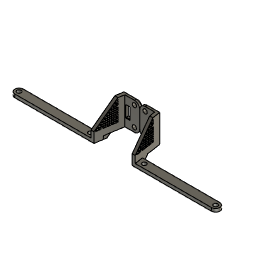
BLTouch_Halter_standardv4 (Autodesk Fusion 360 design; units mm, degrees)
Autodesk Fusion 360 part; units mm, degrees
note: some values were not read from the file. Chosen so that the rebuilt part matches the saved one: which face or edge a step refers to.
(part 1 of 2)
sketch "Skizze1" plane through (0, 0, 0) normal (0, 0, 1) x (1, 0, 0)
  line L0 (115.7718, 101.7058) -> (145.7718, 101.7066) construction
  line L1 (93.7718, 101.7055) -> (63.7718, 101.7055) construction
  line L2 (63.7718, 101.7055) -> (71.2754, 51.2606) construction
  line L3 (145.7718, 101.7066) -> (138.2754, 51.2606) construction
  circle A0 centre (63.7718, 101.7055) radius 1.5
  circle A1 centre (145.7718, 101.7066) radius 1.5
  circle A2 centre (138.2754, 51.2606) radius 2
  circle A3 centre (71.2754, 51.2606) radius 2
  circle A4 centre (93.7718, 101.7055) radius 1.5
  circle A5 centre (115.7718, 101.7058) radius 1.5
  line L4 (145.7718, 101.7066) -> (108.2713, 130.0389) construction
  line L5 (108.2713, 130.0389) -> (101.2713, 130.0389) construction
  line L6 (101.2713, 130.0389) -> (63.7718, 101.7055) construction
  circle A6 centre (101.2713, 130.0389) radius 1
  circle A7 centre (108.2713, 130.0389) radius 1
  line L7 (103.2307, 127.4457) -> (106.3121, 127.4456)
  line L8 (71.2754, 51.2606) -> (71.2754, 46.4951) construction
  line L9 (71.2754, 51.2606) -> (69.2754, 51.2606) construction
  line L10 (71.2754, 51.2606) -> (138.2754, 51.2606) construction
  line L11 (143.9247, 55.2606) -> (146.8968, 75.2606)
  line L12 (71.2754, 47.2606) -> (138.2754, 47.2606)
  arc A8 (138.8634, 55.2171) -> (138.2754, 55.2606) centre (138.2754, 51.2606) ccw
  line L13 (138.2754, 55.2606) -> (71.2754, 55.2606)
  arc A9 (71.2754, 55.2606) -> (71.2754, 47.2606) centre (71.2754, 51.2606) ccw
  line L14 (71.2754, 51.2606) -> (138.2754, 51.2606) construction
  line L15 (138.2754, 55.2606) -> (143.9247, 55.2606)
  line L16 (146.8968, 75.2606) -> (163.4839, 75.2606)
  line L17 (163.4839, 75.2606) -> (163.4839, 72.2606)
  line L18 (163.4839, 72.2606) -> (149.4839, 72.2606)
  line L19 (149.4839, 72.2606) -> (145.5714, 47.2606)
  line L20 (138.2754, 47.2606) -> (145.5714, 47.2606)
  line L21 (143.9247, 55.2606) -> (142.7359, 47.2606) construction
  line L22 (149.4839, 72.2606) -> (149.4839, 75.2606) construction
  dimension "d8" = 30
  dimension "d9" = 30
  dimension "d11" = 3
  dimension "d12" = 3
  dimension "d13" = 4
  dimension "d14" = 4
  dimension "d16" = 51
  dimension "d17" = 81.546
  dimension "d19" = 81.5
  dimension "d28" = 3
  dimension "d29" = 3
  dimension "d30" = 47
  dimension "d31" = 47
  dimension "d33" = 7
  dimension "d34" = 2
  dimension "d35" = 2
  dimension "d36" = 37.1
  dimension "d37" = 142.9
  dimension "d38" = 37.1
  dimension "d39" = 67
  dimension "d69" = 8
  dimension "d71" = 5
  dimension "d73" = 24
  dimension "d74" = 3
  dimension "d75" = 3
  dimension "d76" = 14
  constraint horizontal L1
  constraint coincident L1.end L2.start
  constraint coincident L0.end L3.start
  constraint coincident L3.end A2.centre
  constraint coincident L2.end A3.centre
  constraint coincident L1.start A4.centre
  constraint coincident L0.start A5.centre
  constraint horizontal L5
  constraint coincident L5.end L6.start
  constraint coincident L4.end L5.start
  constraint perpendicular L8 L9
  constraint coincident A3 L9.end
  constraint perpendicular L8 L10
  constraint parallel L3 L11
  constraint tangent L12 A8
  constraint tangent A8 L13
  constraint parallel L12 L13
  constraint tangent L13 A9
  constraint tangent L12 A9
  constraint parallel L10 L14
  constraint tangent A8 L15
  constraint coincident L3 A8.start
  constraint horizontal L16
  constraint perpendicular L16 L17
  constraint perpendicular L17 L18
  constraint parallel L12 L20
  constraint coincident L20 L21.end
  constraint parallel L11 L21
  constraint coincident L16 L22.end
  constraint perpendicular L16 L22
  measures "d8" distance of L0.start L0.end
  measures "d9" distance of L1.start L1.end
  measures "d11" diameter of A0
  measures "d12" diameter of A1
  measures "d13" diameter of A2
  measures "d14" diameter of A3
  measures "d16" distance of L3.end L0.end
  measures "d17" angle of L0 L3
  measures "d28" diameter of A4
  measures "d29" diameter of A5
  measures "d30" distance of L0.end L4.end
  measures "d31" distance of L5.end L1.end
  measures "d33" distance of L4.end L5.end
  measures "d34" diameter of A6
  measures "d35" diameter of A7
  measures "d39" distance of L2.end L3.end
  measures "d69" diameter of A8
  measures "d71" distance of L3 L11
  measures "d73" vertical distance of L3.end L11.end
  measures "d74" distance of L16.end L17.end
  measures "d75" distance of L11 L18.end
  measures "d76" distance of L17.end L18.end
extrude "Extrusion11" add sketch "Skizze1" along normal blind 3 contours L11 L12 L13 A9 L15 L16 L17 L18 L19 L20 makes body 1
sketch "Skizze8" plane through (0, 0, 3) normal (0, 0, 1) x (-1, 0, 0)
  circle A0 centre (-138.2754, -51.2606) radius 2
  circle A1 centre (-71.2754, -51.2606) radius 2
  line L0 (-143.9247, -55.2606) -> (-71.2754, -55.2606)
  arc A2 (-71.2754, -55.2606) -> (-71.2754, -47.2606) centre (-71.2754, -51.2606) ccw
  line L1 (-71.2754, -47.2606) -> (-145.5714, -47.2606)
  line L2 (-145.5714, -47.2606) -> (-149.4839, -72.2606)
  line L3 (-149.4839, -72.2606) -> (-163.4839, -72.2606)
  line L4 (-163.4839, -72.2606) -> (-163.4839, -75.2606)
  line L5 (-163.4839, -75.2606) -> (-146.8968, -75.2606)
  line L6 (-146.8968, -75.2606) -> (-143.9247, -55.2606)
  line L7 (-143.9247, -55.2606) -> (-142.7359, -47.2606)
  line L8 (-143.9247, -55.2606) -> (-146.8968, -75.2606)
  line L9 (-163.4839, -75.2606) -> (-163.4839, -72.2606)
  line L10 (-149.4839, -72.2606) -> (-163.4839, -72.2606)
  line L11 (-149.4839, -72.2606) -> (-145.5714, -47.2606)
  line L12 (-145.5714, -47.2606) -> (-142.7359, -47.2606)
  constraint coincident L0.start L6.end
  constraint coincident L1 L7.end
  constraint parallel L6 L7
  constraint coincident L5.end L6.start
  constraint coincident L4.end L5.start
  constraint coincident L3.end L4.start
  constraint coincident L2.end L3.start
  constraint coincident L1.end L2.start
extrude "Extrusion12" add sketch "Skizze8" along normal blind 23 contours L1 L2 L3 L4 L5 L6 L7 L8 L9 L10 L11 L12 bodies 1
sketch "Skizze10" plane through (0, 75.2606, 0) normal (0, 1, 0) x (-1, 0, 0)
  line L0 (-163.4839, 0) -> (-146.8968, 0)
  line L1 (-146.8968, 0) -> (-146.8968, 26)
  line L2 (-146.8968, 26) -> (-163.4839, 26)
  line L3 (-163.4839, 26) -> (-163.4839, 0)
  line L4 (-158.4839, 26) -> (-158.4839, 0) construction
  line L5 (-146.8968, 13) -> (-163.4839, 13) construction
  circle A0 centre (-158.4839, 22) radius 2
  circle A1 centre (-158.4839, 4) radius 2
  point P0 (-158.4839, 13)
  dimension "d82" = 4
  dimension "d83" = 9
  dimension "d111" = 5
  dimension "d112" = 9
  constraint midpoint L1 L5.start
  constraint midpoint L3 L5.end
  constraint coincident L4 A0.centre
  constraint coincident L4 A1.centre
  measures "d82" diameter of A0
  measures "d83" distance of P0 A0.centre
  measures "d111" distance of L3 L4
  measures "d112" distance of L5 A1.centre
extrude "Extrusion13" cut sketch "Skizze10" against normal blind 6 contours A0 | A1 bodies 1
fillet "Abrundung1" radius 5 2 edges at (163.4839, 73.7606, 26) (163.4839, 73.7606, 0) on bodies 1
chamfer "Fase1" distance 19.5 angle 45 1 edges at (144.1537, 47.2606, 26) on bodies 1
sketch "Skizze12" plane through (132.7809, -19.7314, 0) normal (-0.989138, 0.146987, 0) x (-0.146987, -0.989138, 0)
  line L0 (-67.7276, 6.5) -> (-87.4417, 26)
  line L1 (-87.4417, 26) -> (-96.035, 26)
  line L2 (-96.035, 26) -> (-96.035, 0)
  line L3 (-96.035, 0) -> (-75.8154, 0)
  line L4 (-75.8154, 0) -> (-75.8154, 3)
  line L5 (-75.8154, 3) -> (-67.7276, 3)
  line L6 (-67.7276, 3) -> (-67.7276, 6.5)
  line L7 (-75.8154, 3) -> (-96.035, 3)
  line L8 (-96.035, 26) -> (-96.035, 3)
  line L9 (-96.035, 26) -> (-87.4417, 26)
  line L10 (-87.4417, 26) -> (-67.7276, 6.5)
  line L11 (-67.7276, 3) -> (-67.7276, 6.5)
  line L12 (-67.7276, 3) -> (-75.8154, 3)
  line L13 (-71.9936, 6) -> (-75.3099, 6)
  line L14 (-75.3099, 6) -> (-87.9801, 6)
  line L15 (-87.9801, 21.8129) -> (-87.9801, 6)
  line L16 (-87.6401, 24.2897) -> (-69.5914, 6.437)
  line L17 (-87.9801, 21.8129) -> (-87.9801, 24.2897)
  line L18 (-71.9936, 6) -> (-69.5914, 6)
  line L19 (-69.5914, 6) -> (-69.5914, 6.437)
  line L20 (-87.9801, 24.2897) -> (-87.9472, 24.2897)
  line L21 (-87.9472, 24.2897) -> (-87.6401, 24.2897)
  line L22 (-75.8154, 1.0103) -> (-75.3808, 0.584)
  line L23 (-74.6486, 3) -> (-73.8108, 2.1712)
  line L24 (-79.7376, 15.0605) -> (-80.8491, 14.7474)
  line L25 (-80.8491, 14.7474) -> (-81.1336, 13.6283)
  line L26 (-81.1336, 13.6283) -> (-80.3068, 12.8223)
  line L27 (-80.3068, 12.8223) -> (-79.1953, 13.1355)
  line L28 (-79.1953, 13.1355) -> (-78.9108, 14.2545)
  line L29 (-78.9108, 14.2545) -> (-79.7376, 15.0605)
  line L30 (-97.415, 14.964) -> (-98.5265, 14.6509)
  line L31 (-98.5265, 14.6509) -> (-98.811, 13.5318)
  line L32 (-98.811, 13.5318) -> (-97.9842, 12.7258)
  line L33 (-97.9842, 12.7258) -> (-96.8727, 13.0389)
  line L34 (-96.5882, 14.158) -> (-97.415, 14.964)
  line L35 (-96.8727, 13.0389) -> (-96.5882, 14.158)
  line L36 (-95.6377, 13.2059) -> (-96.7491, 12.8928)
  line L37 (-96.7491, 12.8928) -> (-97.0336, 11.7737)
  line L38 (-97.0336, 11.7737) -> (-96.2068, 10.9677)
  line L39 (-96.2068, 10.9677) -> (-95.0953, 11.2808)
  line L40 (-94.8108, 12.3999) -> (-95.6377, 13.2059)
  line L41 (-95.0953, 11.2808) -> (-94.8108, 12.3999)
  line L42 (-93.8603, 11.4478) -> (-94.9717, 11.1347)
  line L43 (-94.9717, 11.1347) -> (-95.2563, 10.0156)
  line L44 (-95.2563, 10.0156) -> (-94.4294, 9.2096)
  line L45 (-94.4294, 9.2096) -> (-93.3179, 9.5228)
  line L46 (-93.0334, 10.6418) -> (-93.8603, 11.4478)
  line L47 (-93.3179, 9.5228) -> (-93.0334, 10.6418)
  line L48 (-92.0829, 9.6897) -> (-93.1943, 9.3766)
  line L49 (-93.1943, 9.3766) -> (-93.4789, 8.2575)
  line L50 (-93.4789, 8.2575) -> (-92.652, 7.4516)
  line L51 (-92.652, 7.4516) -> (-91.5405, 7.7647)
  line L52 (-91.256, 8.8838) -> (-92.0829, 9.6897)
  line L53 (-91.5405, 7.7647) -> (-91.256, 8.8838)
  line L54 (-90.3055, 7.9316) -> (-91.4169, 7.6185)
  line L55 (-91.4169, 7.6185) -> (-91.7015, 6.4994)
  line L56 (-91.7015, 6.4994) -> (-90.8746, 5.6935)
  line L57 (-90.8746, 5.6935) -> (-89.7631, 6.0066)
  line L58 (-89.4786, 7.1257) -> (-90.3055, 7.9316)
  line L59 (-89.7631, 6.0066) -> (-89.4786, 7.1257)
  line L60 (-88.5281, 6.1736) -> (-89.6395, 5.8604)
  line L61 (-89.6395, 5.8604) -> (-89.9241, 4.7414)
  line L62 (-89.9241, 4.7414) -> (-89.0972, 3.9354)
  line L63 (-89.0972, 3.9354) -> (-87.9858, 4.2485)
  line L64 (-87.7012, 5.3676) -> (-88.5281, 6.1736)
  line L65 (-87.9858, 4.2485) -> (-87.7012, 5.3676)
  line L66 (-86.7507, 4.4155) -> (-87.8621, 4.1024)
  line L67 (-87.8621, 4.1024) -> (-88.1467, 2.9833)
  line L68 (-88.1467, 2.9833) -> (-87.3198, 2.1773)
  line L69 (-87.3198, 2.1773) -> (-86.2084, 2.4904)
  line L70 (-85.9238, 3.6095) -> (-86.7507, 4.4155)
  line L71 (-86.2084, 2.4904) -> (-85.9238, 3.6095)
  line L72 (-84.9733, 2.6574) -> (-86.0847, 2.3443)
  line L73 (-86.0847, 2.3443) -> (-86.3693, 1.2252)
  line L74 (-86.3693, 1.2252) -> (-85.5424, 0.4192)
  line L75 (-85.5424, 0.4192) -> (-84.431, 0.7323)
  line L76 (-84.1464, 1.8514) -> (-84.9733, 2.6574)
  line L77 (-84.431, 0.7323) -> (-84.1464, 1.8514)
  line L78 (-83.1959, 0.8993) -> (-84.3073, 0.5862)
  line L79 (-84.3073, 0.5862) -> (-84.5919, -0.5329)
  line L80 (-84.5919, -0.5329) -> (-83.765, -1.3389)
  line L81 (-83.765, -1.3389) -> (-82.6536, -1.0258)
  line L82 (-82.369, 0.0933) -> (-83.1959, 0.8993)
  line L83 (-82.6536, -1.0258) -> (-82.369, 0.0933)
  line L84 (-81.4185, -0.8588) -> (-82.5299, -1.1719)
  line L85 (-82.5299, -1.1719) -> (-82.8145, -2.291)
  line L86 (-82.8145, -2.291) -> (-81.9876, -3.097)
  line L87 (-81.9876, -3.097) -> (-80.8762, -2.7839)
  line L88 (-80.5916, -1.6648) -> (-81.4185, -0.8588)
  line L89 (-80.8762, -2.7839) -> (-80.5916, -1.6648)
  line L90 (-79.6411, -2.6169) -> (-80.7526, -2.93)
  line L91 (-80.7526, -2.93) -> (-81.0371, -4.0491)
  line L92 (-81.0371, -4.0491) -> (-80.2102, -4.8551)
  line L93 (-80.2102, -4.8551) -> (-79.0988, -4.5419)
  line L94 (-78.8142, -3.4229) -> (-79.6411, -2.6169)
  line L95 (-79.0988, -4.5419) -> (-78.8142, -3.4229)
  line L96 (-95.657, 16.7414) -> (-96.7684, 16.4283)
  line L97 (-96.7684, 16.4283) -> (-97.053, 15.3092)
  line L98 (-97.053, 15.3092) -> (-96.2261, 14.5032)
  line L99 (-96.2261, 14.5032) -> (-95.1146, 14.8163)
  line L100 (-94.8301, 15.9354) -> (-95.657, 16.7414)
  line L101 (-95.1146, 14.8163) -> (-94.8301, 15.9354)
  line L102 (-93.8796, 14.9833) -> (-94.991, 14.6702)
  line L103 (-94.991, 14.6702) -> (-95.2756, 13.5511)
  line L104 (-95.2756, 13.5511) -> (-94.4487, 12.7451)
  line L105 (-94.4487, 12.7451) -> (-93.3372, 13.0582)
  line L106 (-93.0527, 14.1773) -> (-93.8796, 14.9833)
  line L107 (-93.3372, 13.0582) -> (-93.0527, 14.1773)
  line L108 (-92.1022, 13.2252) -> (-93.2136, 12.9121)
  line L109 (-93.2136, 12.9121) -> (-93.4982, 11.793)
  line L110 (-93.4982, 11.793) -> (-92.6713, 10.987)
  line L111 (-92.6713, 10.987) -> (-91.5598, 11.3001)
  line L112 (-91.2753, 12.4192) -> (-92.1022, 13.2252)
  line L113 (-91.5598, 11.3001) -> (-91.2753, 12.4192)
  line L114 (-90.3248, 11.4671) -> (-91.4362, 11.154)
  line L115 (-91.4362, 11.154) -> (-91.7208, 10.0349)
  line L116 (-91.7208, 10.0349) -> (-90.8939, 9.2289)
  line L117 (-90.8939, 9.2289) -> (-89.7825, 9.5421)
  line L118 (-89.4979, 10.6612) -> (-90.3248, 11.4671)
  line L119 (-89.7825, 9.5421) -> (-89.4979, 10.6612)
  line L120 (-88.5474, 9.709) -> (-89.6588, 9.3959)
  line L121 (-89.6588, 9.3959) -> (-89.9434, 8.2768)
  line L122 (-89.9434, 8.2768) -> (-89.1165, 7.4709)
  line L123 (-89.1165, 7.4709) -> (-88.0051, 7.784)
  line L124 (-87.7205, 8.9031) -> (-88.5474, 9.709)
  line L125 (-88.0051, 7.784) -> (-87.7205, 8.9031)
  line L126 (-86.77, 7.951) -> (-87.8814, 7.6378)
  line L127 (-87.8814, 7.6378) -> (-88.166, 6.5187)
  line L128 (-88.166, 6.5187) -> (-87.3391, 5.7128)
  line L129 (-87.3391, 5.7128) -> (-86.2277, 6.0259)
  line L130 (-85.9431, 7.145) -> (-86.77, 7.951)
  line L131 (-86.2277, 6.0259) -> (-85.9431, 7.145)
  line L132 (-84.9926, 6.1929) -> (-86.104, 5.8798)
  line L133 (-86.104, 5.8798) -> (-86.3886, 4.7607)
  line L134 (-86.3886, 4.7607) -> (-85.5617, 3.9547)
  line L135 (-85.5617, 3.9547) -> (-84.4503, 4.2678)
  line L136 (-84.1657, 5.3869) -> (-84.9926, 6.1929)
  line L137 (-84.4503, 4.2678) -> (-84.1657, 5.3869)
  line L138 (-83.2152, 4.4348) -> (-84.3266, 4.1217)
  line L139 (-84.3266, 4.1217) -> (-84.6112, 3.0026)
  line L140 (-84.6112, 3.0026) -> (-83.7843, 2.1966)
  line L141 (-83.7843, 2.1966) -> (-82.6729, 2.5097)
  line L142 (-82.3883, 3.6288) -> (-83.2152, 4.4348)
  line L143 (-82.6729, 2.5097) -> (-82.3883, 3.6288)
  line L144 (-81.4378, 2.6767) -> (-82.5493, 2.3636)
  line L145 (-82.5493, 2.3636) -> (-82.8338, 1.2445)
  line L146 (-82.8338, 1.2445) -> (-82.0069, 0.4385)
  line L147 (-82.0069, 0.4385) -> (-80.8955, 0.7516)
  line L148 (-80.6109, 1.8707) -> (-81.4378, 2.6767)
  line L149 (-80.8955, 0.7516) -> (-80.6109, 1.8707)
  line L150 (-79.6604, 0.9186) -> (-80.7719, 0.6055)
  line L151 (-80.7719, 0.6055) -> (-81.0564, -0.5136)
  line L152 (-81.0564, -0.5136) -> (-80.2295, -1.3196)
  line L153 (-80.2295, -1.3196) -> (-79.1181, -1.0065)
  line L154 (-78.8335, 0.1126) -> (-79.6604, 0.9186)
  line L155 (-79.1181, -1.0065) -> (-78.8335, 0.1126)
  line L156 (-77.883, -0.8395) -> (-78.9945, -1.1526)
  line L157 (-78.9945, -1.1526) -> (-79.279, -2.2717)
  line L158 (-79.279, -2.2717) -> (-78.4521, -3.0777)
  line L159 (-78.4521, -3.0777) -> (-77.3407, -2.7646)
  line L160 (-77.0561, -1.6455) -> (-77.883, -0.8395)
  line L161 (-77.3407, -2.7646) -> (-77.0561, -1.6455)
  line L162 (-93.8989, 18.5188) -> (-95.0103, 18.2057)
  line L163 (-95.0103, 18.2057) -> (-95.2949, 17.0866)
  line L164 (-95.2949, 17.0866) -> (-94.468, 16.2806)
  line L165 (-94.468, 16.2806) -> (-93.3565, 16.5937)
  line L166 (-93.072, 17.7128) -> (-93.8989, 18.5188)
  line L167 (-93.3565, 16.5937) -> (-93.072, 17.7128)
  line L168 (-92.1215, 16.7607) -> (-93.2329, 16.4476)
  line L169 (-93.2329, 16.4476) -> (-93.5175, 15.3285)
  line L170 (-93.5175, 15.3285) -> (-92.6906, 14.5225)
  line L171 (-92.6906, 14.5225) -> (-91.5792, 14.8356)
  line L172 (-91.2946, 15.9547) -> (-92.1215, 16.7607)
  line L173 (-91.5792, 14.8356) -> (-91.2946, 15.9547)
  line L174 (-90.3441, 15.0026) -> (-91.4555, 14.6895)
  line L175 (-91.4555, 14.6895) -> (-91.7401, 13.5704)
  line L176 (-91.7401, 13.5704) -> (-90.9132, 12.7644)
  line L177 (-90.9132, 12.7644) -> (-89.8018, 13.0775)
  line L178 (-89.5172, 14.1966) -> (-90.3441, 15.0026)
  line L179 (-89.8018, 13.0775) -> (-89.5172, 14.1966)
  line L180 (-88.5667, 13.2445) -> (-89.6781, 12.9314)
  line L181 (-89.6781, 12.9314) -> (-89.9627, 11.8123)
  line L182 (-89.9627, 11.8123) -> (-89.1358, 11.0063)
  line L183 (-89.1358, 11.0063) -> (-88.0244, 11.3195)
  line L184 (-87.7398, 12.4385) -> (-88.5667, 13.2445)
  line L185 (-88.0244, 11.3195) -> (-87.7398, 12.4385)
  line L186 (-86.7893, 11.4864) -> (-87.9007, 11.1733)
  line L187 (-87.9007, 11.1733) -> (-88.1853, 10.0542)
  line L188 (-88.1853, 10.0542) -> (-87.3584, 9.2483)
  line L189 (-87.3584, 9.2483) -> (-86.247, 9.5614)
  line L190 (-85.9624, 10.6805) -> (-86.7893, 11.4864)
  line L191 (-86.247, 9.5614) -> (-85.9624, 10.6805)
  line L192 (-85.0119, 9.7283) -> (-86.1233, 9.4152)
  line L193 (-86.1233, 9.4152) -> (-86.4079, 8.2961)
  line L194 (-86.4079, 8.2961) -> (-85.581, 7.4902)
  line L195 (-85.581, 7.4902) -> (-84.4696, 7.8033)
  line L196 (-84.185, 8.9224) -> (-85.0119, 9.7283)
  line L197 (-84.4696, 7.8033) -> (-84.185, 8.9224)
  line L198 (-83.2345, 7.9703) -> (-84.3459, 7.6571)
  line L199 (-84.3459, 7.6571) -> (-84.6305, 6.5381)
  line L200 (-84.6305, 6.5381) -> (-83.8036, 5.7321)
  line L201 (-83.8036, 5.7321) -> (-82.6922, 6.0452)
  line L202 (-82.4076, 7.1643) -> (-83.2345, 7.9703)
  line L203 (-82.6922, 6.0452) -> (-82.4076, 7.1643)
  line L204 (-81.4571, 6.2122) -> (-82.5686, 5.8991)
  line L205 (-82.5686, 5.8991) -> (-82.8531, 4.78)
  line L206 (-82.8531, 4.78) -> (-82.0262, 3.974)
  line L207 (-82.0262, 3.974) -> (-80.9148, 4.2871)
  line L208 (-80.6302, 5.4062) -> (-81.4571, 6.2122)
  line L209 (-80.9148, 4.2871) -> (-80.6302, 5.4062)
  line L210 (-79.6797, 4.4541) -> (-80.7912, 4.141)
  line L211 (-80.7912, 4.141) -> (-81.0757, 3.0219)
  line L212 (-81.0757, 3.0219) -> (-80.2488, 2.2159)
  line L213 (-80.2488, 2.2159) -> (-79.1374, 2.529)
  line L214 (-78.8528, 3.6481) -> (-79.6797, 4.4541)
  line L215 (-79.1374, 2.529) -> (-78.8528, 3.6481)
  line L216 (-77.9023, 2.696) -> (-79.0138, 2.3829)
  line L217 (-79.0138, 2.3829) -> (-79.2983, 1.2638)
  line L218 (-79.2983, 1.2638) -> (-78.4714, 0.4578)
  line L219 (-78.4714, 0.4578) -> (-77.36, 0.7709)
  line L220 (-77.0755, 1.89) -> (-77.9023, 2.696)
  line L221 (-77.36, 0.7709) -> (-77.0755, 1.89)
  line L222 (-76.1249, 0.9379) -> (-77.2364, 0.6248)
  line L223 (-77.2364, 0.6248) -> (-77.5209, -0.4943)
  line L224 (-77.5209, -0.4943) -> (-76.6941, -1.3003)
  line L225 (-76.6941, -1.3003) -> (-75.5826, -0.9872)
  line L226 (-75.2981, 0.1319) -> (-76.1249, 0.9379)
  line L227 (-75.5826, -0.9872) -> (-75.2981, 0.1319)
  line L228 (-92.1408, 20.2962) -> (-93.2522, 19.9831)
  line L229 (-93.2522, 19.9831) -> (-93.5368, 18.864)
  line L230 (-93.5368, 18.864) -> (-92.7099, 18.058)
  line L231 (-92.7099, 18.058) -> (-91.5985, 18.3711)
  line L232 (-91.3139, 19.4902) -> (-92.1408, 20.2962)
  line L233 (-91.5985, 18.3711) -> (-91.3139, 19.4902)
  line L234 (-90.3634, 18.5381) -> (-91.4748, 18.225)
  line L235 (-91.4748, 18.225) -> (-91.7594, 17.1059)
  line L236 (-91.7594, 17.1059) -> (-90.9325, 16.2999)
  line L237 (-90.9325, 16.2999) -> (-89.8211, 16.613)
  line L238 (-89.5365, 17.7321) -> (-90.3634, 18.5381)
  line L239 (-89.8211, 16.613) -> (-89.5365, 17.7321)
  line L240 (-88.586, 16.78) -> (-89.6974, 16.4669)
  line L241 (-89.6974, 16.4669) -> (-89.982, 15.3478)
  line L242 (-89.982, 15.3478) -> (-89.1551, 14.5418)
  line L243 (-89.1551, 14.5418) -> (-88.0437, 14.8549)
  line L244 (-87.7591, 15.974) -> (-88.586, 16.78)
  line L245 (-88.0437, 14.8549) -> (-87.7591, 15.974)
  line L246 (-86.8086, 15.0219) -> (-87.92, 14.7088)
  line L247 (-87.92, 14.7088) -> (-88.2046, 13.5897)
  line L248 (-88.2046, 13.5897) -> (-87.3777, 12.7837)
  line L249 (-87.3777, 12.7837) -> (-86.2663, 13.0968)
  line L250 (-85.9817, 14.2159) -> (-86.8086, 15.0219)
  line L251 (-86.2663, 13.0968) -> (-85.9817, 14.2159)
  line L252 (-85.0312, 13.2638) -> (-86.1426, 12.9507)
  line L253 (-86.1426, 12.9507) -> (-86.4272, 11.8316)
  line L254 (-86.4272, 11.8316) -> (-85.6003, 11.0256)
  line L255 (-85.6003, 11.0256) -> (-84.4889, 11.3388)
  line L256 (-84.2043, 12.4578) -> (-85.0312, 13.2638)
  line L257 (-84.4889, 11.3388) -> (-84.2043, 12.4578)
  line L258 (-83.2538, 11.5057) -> (-84.3653, 11.1926)
  line L259 (-84.3653, 11.1926) -> (-84.6498, 10.0735)
  line L260 (-84.6498, 10.0735) -> (-83.8229, 9.2676)
  line L261 (-83.8229, 9.2676) -> (-82.7115, 9.5807)
  line L262 (-82.4269, 10.6998) -> (-83.2538, 11.5057)
  line L263 (-82.7115, 9.5807) -> (-82.4269, 10.6998)
  line L264 (-81.4764, 9.7477) -> (-82.5879, 9.4345)
  line L265 (-82.5879, 9.4345) -> (-82.8724, 8.3154)
  line L266 (-82.8724, 8.3154) -> (-82.0455, 7.5095)
  line L267 (-82.0455, 7.5095) -> (-80.9341, 7.8226)
  line L268 (-80.6495, 8.9417) -> (-81.4764, 9.7477)
  line L269 (-80.9341, 7.8226) -> (-80.6495, 8.9417)
  line L270 (-79.699, 7.9896) -> (-80.8105, 7.6765)
  line L271 (-80.8105, 7.6765) -> (-81.095, 6.5574)
  line L272 (-81.095, 6.5574) -> (-80.2681, 5.7514)
  line L273 (-80.2681, 5.7514) -> (-79.1567, 6.0645)
  line L274 (-78.8721, 7.1836) -> (-79.699, 7.9896)
  line L275 (-79.1567, 6.0645) -> (-78.8721, 7.1836)
  line L276 (-77.9216, 6.2315) -> (-79.0331, 5.9184)
  line L277 (-79.0331, 5.9184) -> (-79.3176, 4.7993)
  line L278 (-79.3176, 4.7993) -> (-78.4907, 3.9933)
  line L279 (-78.4907, 3.9933) -> (-77.3793, 4.3064)
  line L280 (-77.0948, 5.4255) -> (-77.9216, 6.2315)
  line L281 (-77.3793, 4.3064) -> (-77.0948, 5.4255)
  line L282 (-76.1442, 4.4734) -> (-77.2557, 4.1603)
  line L283 (-77.2557, 4.1603) -> (-77.5402, 3.0412)
  line L284 (-77.5402, 3.0412) -> (-76.7134, 2.2352)
  line L285 (-76.7134, 2.2352) -> (-75.6019, 2.5483)
  line L286 (-75.3174, 3.6674) -> (-76.1442, 4.4734)
  line L287 (-75.6019, 2.5483) -> (-75.3174, 3.6674)
  line L288 (-74.3669, 2.7153) -> (-75.4783, 2.4022)
  line L289 (-75.4783, 2.4022) -> (-75.7628, 1.2831)
  line L290 (-75.7628, 1.2831) -> (-74.936, 0.4771)
  line L291 (-74.936, 0.4771) -> (-73.8245, 0.7902)
  line L292 (-73.54, 1.9093) -> (-74.3669, 2.7153)
  line L293 (-73.8245, 0.7902) -> (-73.54, 1.9093)
  line L294 (-90.3827, 22.0736) -> (-91.4941, 21.7605)
  line L295 (-91.4941, 21.7605) -> (-91.7787, 20.6414)
  line L296 (-91.7787, 20.6414) -> (-90.9518, 19.8354)
  line L297 (-90.9518, 19.8354) -> (-89.8404, 20.1485)
  line L298 (-89.5558, 21.2676) -> (-90.3827, 22.0736)
  line L299 (-89.8404, 20.1485) -> (-89.5558, 21.2676)
  line L300 (-88.6053, 20.3155) -> (-89.7167, 20.0024)
  line L301 (-89.7167, 20.0024) -> (-90.0013, 18.8833)
  line L302 (-90.0013, 18.8833) -> (-89.1744, 18.0773)
  line L303 (-89.1744, 18.0773) -> (-88.063, 18.3904)
  line L304 (-87.7784, 19.5095) -> (-88.6053, 20.3155)
  line L305 (-88.063, 18.3904) -> (-87.7784, 19.5095)
  line L306 (-86.8279, 18.5574) -> (-87.9393, 18.2443)
  line L307 (-87.9393, 18.2443) -> (-88.2239, 17.1252)
  line L308 (-88.2239, 17.1252) -> (-87.397, 16.3192)
  line L309 (-87.397, 16.3192) -> (-86.2856, 16.6323)
  line L310 (-86.001, 17.7514) -> (-86.8279, 18.5574)
  line L311 (-86.2856, 16.6323) -> (-86.001, 17.7514)
  line L312 (-85.0505, 16.7993) -> (-86.162, 16.4862)
  line L313 (-86.162, 16.4862) -> (-86.4465, 15.3671)
  line L314 (-86.4465, 15.3671) -> (-85.6196, 14.5611)
  line L315 (-85.6196, 14.5611) -> (-84.5082, 14.8742)
  line L316 (-84.2236, 15.9933) -> (-85.0505, 16.7993)
  line L317 (-84.5082, 14.8742) -> (-84.2236, 15.9933)
  line L318 (-83.2731, 15.0412) -> (-84.3846, 14.7281)
  line L319 (-84.3846, 14.7281) -> (-84.6691, 13.609)
  line L320 (-84.6691, 13.609) -> (-83.8422, 12.803)
  line L321 (-83.8422, 12.803) -> (-82.7308, 13.1162)
  line L322 (-82.4462, 14.2352) -> (-83.2731, 15.0412)
  line L323 (-82.7308, 13.1162) -> (-82.4462, 14.2352)
  line L324 (-81.4957, 13.2831) -> (-82.6072, 12.97)
  line L325 (-82.6072, 12.97) -> (-82.8917, 11.8509)
  line L326 (-82.8917, 11.8509) -> (-82.0648, 11.045)
  line L327 (-82.0648, 11.045) -> (-80.9534, 11.3581)
  line L328 (-80.6688, 12.4772) -> (-81.4957, 13.2831)
  line L329 (-80.9534, 11.3581) -> (-80.6688, 12.4772)
  line L330 (-79.7183, 11.525) -> (-80.8298, 11.2119)
  line L331 (-80.8298, 11.2119) -> (-81.1143, 10.0928)
  line L332 (-81.1143, 10.0928) -> (-80.2874, 9.2869)
  line L333 (-80.2874, 9.2869) -> (-79.176, 9.6)
  line L334 (-78.8915, 10.7191) -> (-79.7183, 11.525)
  line L335 (-79.176, 9.6) -> (-78.8915, 10.7191)
  line L336 (-77.9409, 9.767) -> (-79.0524, 9.4538)
  line L337 (-79.0524, 9.4538) -> (-79.3369, 8.3348)
  line L338 (-79.3369, 8.3348) -> (-78.5101, 7.5288)
  line L339 (-78.5101, 7.5288) -> (-77.3986, 7.8419)
  line L340 (-77.1141, 8.961) -> (-77.9409, 9.767)
  line L341 (-77.3986, 7.8419) -> (-77.1141, 8.961)
  line L342 (-76.1635, 8.0089) -> (-77.275, 7.6958)
  line L343 (-77.275, 7.6958) -> (-77.5595, 6.5767)
  line L344 (-77.5595, 6.5767) -> (-76.7327, 5.7707)
  line L345 (-76.7327, 5.7707) -> (-75.6212, 6.0838)
  line L346 (-75.3367, 7.2029) -> (-76.1635, 8.0089)
  line L347 (-75.6212, 6.0838) -> (-75.3367, 7.2029)
  line L348 (-74.3862, 6.2508) -> (-75.4976, 5.9377)
  line L349 (-75.4976, 5.9377) -> (-75.7821, 4.8186)
  line L350 (-75.7821, 4.8186) -> (-74.9553, 4.0126)
  line L351 (-74.9553, 4.0126) -> (-73.8438, 4.3257)
  line L352 (-73.5593, 5.4448) -> (-74.3862, 6.2508)
  line L353 (-73.8438, 4.3257) -> (-73.5593, 5.4448)
  line L354 (-72.6088, 4.4927) -> (-73.7202, 4.1796)
  line L355 (-73.7202, 4.1796) -> (-74.0048, 3.0605)
  line L356 (-74.0048, 3.0605) -> (-73.1779, 2.2545)
  line L357 (-73.1779, 2.2545) -> (-72.0664, 2.5676)
  line L358 (-71.7819, 3.6867) -> (-72.6088, 4.4927)
  line L359 (-72.0664, 2.5676) -> (-71.7819, 3.6867)
  line L360 (-88.6246, 23.851) -> (-89.736, 23.5379)
  line L361 (-89.736, 23.5379) -> (-90.0206, 22.4188)
  line L362 (-90.0206, 22.4188) -> (-89.1937, 21.6128)
  line L363 (-89.1937, 21.6128) -> (-88.0823, 21.9259)
  line L364 (-87.7977, 23.045) -> (-88.6246, 23.851)
  line L365 (-88.0823, 21.9259) -> (-87.7977, 23.045)
  line L366 (-86.8472, 22.0929) -> (-87.9587, 21.7798)
  line L367 (-87.9587, 21.7798) -> (-88.2432, 20.6607)
  line L368 (-88.2432, 20.6607) -> (-87.4163, 19.8547)
  line L369 (-87.4163, 19.8547) -> (-86.3049, 20.1678)
  line L370 (-86.0203, 21.2869) -> (-86.8472, 22.0929)
  line L371 (-86.3049, 20.1678) -> (-86.0203, 21.2869)
  line L372 (-85.0698, 20.3348) -> (-86.1813, 20.0217)
  line L373 (-86.1813, 20.0217) -> (-86.4658, 18.9026)
  line L374 (-86.4658, 18.9026) -> (-85.6389, 18.0966)
  line L375 (-85.6389, 18.0966) -> (-84.5275, 18.4097)
  line L376 (-84.2429, 19.5288) -> (-85.0698, 20.3348)
  line L377 (-84.5275, 18.4097) -> (-84.2429, 19.5288)
  line L378 (-83.2924, 18.5767) -> (-84.4039, 18.2636)
  line L379 (-84.4039, 18.2636) -> (-84.6884, 17.1445)
  line L380 (-84.6884, 17.1445) -> (-83.8615, 16.3385)
  line L381 (-83.8615, 16.3385) -> (-82.7501, 16.6516)
  line L382 (-82.4655, 17.7707) -> (-83.2924, 18.5767)
  line L383 (-82.7501, 16.6516) -> (-82.4655, 17.7707)
  line L384 (-81.515, 16.8186) -> (-82.6265, 16.5055)
  line L385 (-82.6265, 16.5055) -> (-82.911, 15.3864)
  line L386 (-82.911, 15.3864) -> (-82.0841, 14.5804)
  line L387 (-82.0841, 14.5804) -> (-80.9727, 14.8935)
  line L388 (-80.6882, 16.0126) -> (-81.515, 16.8186)
  line L389 (-80.9727, 14.8935) -> (-80.6882, 16.0126)
  line L390 (-77.9602, 13.3024) -> (-79.0717, 12.9893)
  line L391 (-79.0717, 12.9893) -> (-79.3562, 11.8702)
  line L392 (-79.3562, 11.8702) -> (-78.5294, 11.0643)
  line L393 (-78.5294, 11.0643) -> (-77.4179, 11.3774)
  line L394 (-77.1334, 12.4965) -> (-77.9602, 13.3024)
  line L395 (-77.4179, 11.3774) -> (-77.1334, 12.4965)
  line L396 (-76.1829, 11.5443) -> (-77.2943, 11.2312)
  line L397 (-77.2943, 11.2312) -> (-77.5788, 10.1121)
  line L398 (-77.5788, 10.1121) -> (-76.752, 9.3062)
  line L399 (-76.752, 9.3062) -> (-75.6405, 9.6193)
  line L400 (-75.356, 10.7384) -> (-76.1829, 11.5443)
  line L401 (-75.6405, 9.6193) -> (-75.356, 10.7384)
  line L402 (-74.4055, 9.7863) -> (-75.5169, 9.4731)
  line L403 (-75.5169, 9.4731) -> (-75.8015, 8.3541)
  line L404 (-75.8015, 8.3541) -> (-74.9746, 7.5481)
  line L405 (-74.9746, 7.5481) -> (-73.8631, 7.8612)
  line L406 (-73.5786, 8.9803) -> (-74.4055, 9.7863)
  line L407 (-73.8631, 7.8612) -> (-73.5786, 8.9803)
  line L408 (-72.6281, 8.0282) -> (-73.7395, 7.7151)
  line L409 (-73.7395, 7.7151) -> (-74.0241, 6.596)
  line L410 (-74.0241, 6.596) -> (-73.1972, 5.79)
  line L411 (-73.1972, 5.79) -> (-72.0857, 6.1031)
  line L412 (-71.8012, 7.2222) -> (-72.6281, 8.0282)
  line L413 (-72.0857, 6.1031) -> (-71.8012, 7.2222)
  line L414 (-70.8507, 6.2701) -> (-71.9621, 5.957)
  line L415 (-71.9621, 5.957) -> (-72.2467, 4.8379)
  line L416 (-72.2467, 4.8379) -> (-71.4198, 4.0319)
  line L417 (-71.4198, 4.0319) -> (-70.3083, 4.345)
  line L418 (-70.0238, 5.4641) -> (-70.8507, 6.2701)
  line L419 (-70.3083, 4.345) -> (-70.0238, 5.4641)
  line L420 (-86.8665, 25.6284) -> (-87.978, 25.3152)
  line L421 (-87.978, 25.3152) -> (-88.2625, 24.1962)
  line L422 (-88.2625, 24.1962) -> (-87.4356, 23.3902)
  line L423 (-87.4356, 23.3902) -> (-86.3242, 23.7033)
  line L424 (-86.0396, 24.8224) -> (-86.8665, 25.6284)
  line L425 (-86.3242, 23.7033) -> (-86.0396, 24.8224)
  line L426 (-85.0891, 23.8703) -> (-86.2006, 23.5572)
  line L427 (-86.2006, 23.5572) -> (-86.4851, 22.4381)
  line L428 (-86.4851, 22.4381) -> (-85.6582, 21.6321)
  line L429 (-85.6582, 21.6321) -> (-84.5468, 21.9452)
  line L430 (-84.2622, 23.0643) -> (-85.0891, 23.8703)
  line L431 (-84.5468, 21.9452) -> (-84.2622, 23.0643)
  line L432 (-83.3117, 22.1122) -> (-84.4232, 21.7991)
  line L433 (-84.4232, 21.7991) -> (-84.7077, 20.68)
  line L434 (-84.7077, 20.68) -> (-83.8808, 19.874)
  line L435 (-83.8808, 19.874) -> (-82.7694, 20.1871)
  line L436 (-82.4849, 21.3062) -> (-83.3117, 22.1122)
  line L437 (-82.7694, 20.1871) -> (-82.4849, 21.3062)
  line L438 (-81.5343, 20.3541) -> (-82.6458, 20.041)
  line L439 (-82.6458, 20.041) -> (-82.9303, 18.9219)
  line L440 (-82.9303, 18.9219) -> (-82.1035, 18.1159)
  line L441 (-82.1035, 18.1159) -> (-80.992, 18.429)
  line L442 (-80.7075, 19.5481) -> (-81.5343, 20.3541)
  line L443 (-80.992, 18.429) -> (-80.7075, 19.5481)
  line L444 (-79.7569, 18.596) -> (-80.8684, 18.2829)
  line L445 (-80.8684, 18.2829) -> (-81.1529, 17.1638)
  line L446 (-81.1529, 17.1638) -> (-80.3261, 16.3578)
  line L447 (-80.3261, 16.3578) -> (-79.2146, 16.6709)
  line L448 (-78.9301, 17.79) -> (-79.7569, 18.596)
  line L449 (-79.2146, 16.6709) -> (-78.9301, 17.79)
  line L450 (-77.9796, 16.8379) -> (-79.091, 16.5248)
  line L451 (-79.091, 16.5248) -> (-79.3755, 15.4057)
  line L452 (-79.3755, 15.4057) -> (-78.5487, 14.5997)
  line L453 (-78.5487, 14.5997) -> (-77.4372, 14.9129)
  line L454 (-77.1527, 16.0319) -> (-77.9796, 16.8379)
  line L455 (-77.4372, 14.9129) -> (-77.1527, 16.0319)
  line L456 (-76.2022, 15.0798) -> (-77.3136, 14.7667)
  line L457 (-77.3136, 14.7667) -> (-77.5982, 13.6476)
  line L458 (-77.5982, 13.6476) -> (-76.7713, 12.8417)
  line L459 (-76.7713, 12.8417) -> (-75.6598, 13.1548)
  line L460 (-75.3753, 14.2739) -> (-76.2022, 15.0798)
  line L461 (-75.6598, 13.1548) -> (-75.3753, 14.2739)
  line L462 (-74.4248, 13.3217) -> (-75.5362, 13.0086)
  line L463 (-75.5362, 13.0086) -> (-75.8208, 11.8895)
  line L464 (-75.8208, 11.8895) -> (-74.9939, 11.0836)
  line L465 (-74.9939, 11.0836) -> (-73.8824, 11.3967)
  line L466 (-73.5979, 12.5158) -> (-74.4248, 13.3217)
  line L467 (-73.8824, 11.3967) -> (-73.5979, 12.5158)
  line L468 (-72.6474, 11.5637) -> (-73.7588, 11.2505)
  line L469 (-73.7588, 11.2505) -> (-74.0434, 10.1315)
  line L470 (-74.0434, 10.1315) -> (-73.2165, 9.3255)
  line L471 (-73.2165, 9.3255) -> (-72.105, 9.6386)
  line L472 (-71.8205, 10.7577) -> (-72.6474, 11.5637)
  line L473 (-72.105, 9.6386) -> (-71.8205, 10.7577)
  line L474 (-70.87, 9.8056) -> (-71.9814, 9.4925)
  line L475 (-71.9814, 9.4925) -> (-72.266, 8.3734)
  line L476 (-72.266, 8.3734) -> (-71.4391, 7.5674)
  line L477 (-71.4391, 7.5674) -> (-70.3277, 7.8805)
  line L478 (-70.0431, 8.9996) -> (-70.87, 9.8056)
  line L479 (-70.3277, 7.8805) -> (-70.0431, 8.9996)
  line L480 (-69.0926, 8.0475) -> (-70.204, 7.7344)
  line L481 (-70.204, 7.7344) -> (-70.4886, 6.6153)
  line L482 (-70.4886, 6.6153) -> (-69.6617, 5.8093)
  line L483 (-69.6617, 5.8093) -> (-68.5503, 6.1224)
  line L484 (-68.2657, 7.2415) -> (-69.0926, 8.0475)
  line L485 (-68.5503, 6.1224) -> (-68.2657, 7.2415)
  line L486 (-85.1084, 27.4058) -> (-86.2199, 27.0926)
  line L487 (-86.2199, 27.0926) -> (-86.5044, 25.9735)
  line L488 (-86.5044, 25.9735) -> (-85.6775, 25.1676)
  line L489 (-85.6775, 25.1676) -> (-84.5661, 25.4807)
  line L490 (-84.2815, 26.5998) -> (-85.1084, 27.4058)
  line L491 (-84.5661, 25.4807) -> (-84.2815, 26.5998)
  line L492 (-83.331, 25.6477) -> (-84.4425, 25.3346)
  line L493 (-84.4425, 25.3346) -> (-84.727, 24.2155)
  line L494 (-84.727, 24.2155) -> (-83.9001, 23.4095)
  line L495 (-83.9001, 23.4095) -> (-82.7887, 23.7226)
  line L496 (-82.5042, 24.8417) -> (-83.331, 25.6477)
  line L497 (-82.7887, 23.7226) -> (-82.5042, 24.8417)
  line L498 (-81.5536, 23.8896) -> (-82.6651, 23.5765)
  line L499 (-82.6651, 23.5765) -> (-82.9496, 22.4574)
  line L500 (-82.9496, 22.4574) -> (-82.1228, 21.6514)
  line L501 (-82.1228, 21.6514) -> (-81.0113, 21.9645)
  line L502 (-80.7268, 23.0836) -> (-81.5536, 23.8896)
  line L503 (-81.0113, 21.9645) -> (-80.7268, 23.0836)
  line L504 (-79.7763, 22.1315) -> (-80.8877, 21.8184)
  line L505 (-80.8877, 21.8184) -> (-81.1722, 20.6993)
  line L506 (-81.1722, 20.6993) -> (-80.3454, 19.8933)
  line L507 (-80.3454, 19.8933) -> (-79.2339, 20.2064)
  line L508 (-78.9494, 21.3255) -> (-79.7763, 22.1315)
  line L509 (-79.2339, 20.2064) -> (-78.9494, 21.3255)
  line L510 (-77.9989, 20.3734) -> (-79.1103, 20.0603)
  line L511 (-79.1103, 20.0603) -> (-79.3949, 18.9412)
  line L512 (-79.3949, 18.9412) -> (-78.568, 18.1352)
  line L513 (-78.568, 18.1352) -> (-77.4565, 18.4483)
  line L514 (-77.172, 19.5674) -> (-77.9989, 20.3734)
  line L515 (-77.4565, 18.4483) -> (-77.172, 19.5674)
  line L516 (-76.2215, 18.6153) -> (-77.3329, 18.3022)
  line L517 (-77.3329, 18.3022) -> (-77.6175, 17.1831)
  line L518 (-77.6175, 17.1831) -> (-76.7906, 16.3771)
  line L519 (-76.7906, 16.3771) -> (-75.6791, 16.6902)
  line L520 (-75.3946, 17.8093) -> (-76.2215, 18.6153)
  line L521 (-75.6791, 16.6902) -> (-75.3946, 17.8093)
  line L522 (-74.4441, 16.8572) -> (-75.5555, 16.5441)
  line L523 (-75.5555, 16.5441) -> (-75.8401, 15.425)
  line L524 (-75.8401, 15.425) -> (-75.0132, 14.619)
  line L525 (-75.0132, 14.619) -> (-73.9017, 14.9322)
  line L526 (-73.6172, 16.0512) -> (-74.4441, 16.8572)
  line L527 (-73.9017, 14.9322) -> (-73.6172, 16.0512)
  line L528 (-72.6667, 15.0991) -> (-73.7781, 14.786)
  line L529 (-73.7781, 14.786) -> (-74.0627, 13.6669)
  line L530 (-74.0627, 13.6669) -> (-73.2358, 12.861)
  line L531 (-73.2358, 12.861) -> (-72.1244, 13.1741)
  line L532 (-71.8398, 14.2932) -> (-72.6667, 15.0991)
  line L533 (-72.1244, 13.1741) -> (-71.8398, 14.2932)
  line L534 (-70.8893, 13.341) -> (-72.0007, 13.0279)
  line L535 (-72.0007, 13.0279) -> (-72.2853, 11.9088)
  line L536 (-72.2853, 11.9088) -> (-71.4584, 11.1029)
  line L537 (-71.4584, 11.1029) -> (-70.347, 11.416)
  line L538 (-70.0624, 12.5351) -> (-70.8893, 13.341)
  line L539 (-70.347, 11.416) -> (-70.0624, 12.5351)
  line L540 (-69.1119, 11.583) -> (-70.2233, 11.2698)
  line L541 (-70.2233, 11.2698) -> (-70.5079, 10.1508)
  line L542 (-70.5079, 10.1508) -> (-69.681, 9.3448)
  line L543 (-69.681, 9.3448) -> (-68.5696, 9.6579)
  line L544 (-68.285, 10.777) -> (-69.1119, 11.583)
  line L545 (-68.5696, 9.6579) -> (-68.285, 10.777)
  line L546 (-67.3345, 9.8249) -> (-68.4459, 9.5118)
  line L547 (-68.4459, 9.5118) -> (-68.7305, 8.3927)
  line L548 (-68.7305, 8.3927) -> (-67.9036, 7.5867)
  line L549 (-67.9036, 7.5867) -> (-66.7922, 7.8998)
  line L550 (-66.5076, 9.0189) -> (-67.3345, 9.8249)
  line L551 (-66.7922, 7.8998) -> (-66.5076, 9.0189)
  line L552 (-83.3503, 29.1831) -> (-84.4618, 28.87)
  line L553 (-84.4618, 28.87) -> (-84.7463, 27.7509)
  line L554 (-84.7463, 27.7509) -> (-83.9195, 26.945)
  line L555 (-83.9195, 26.945) -> (-82.808, 27.2581)
  line L556 (-82.5235, 28.3772) -> (-83.3503, 29.1831)
  line L557 (-82.808, 27.2581) -> (-82.5235, 28.3772)
  line L558 (-81.573, 27.4251) -> (-82.6844, 27.1119)
  line L559 (-82.6844, 27.1119) -> (-82.9689, 25.9929)
  line L560 (-82.9689, 25.9929) -> (-82.1421, 25.1869)
  line L561 (-82.1421, 25.1869) -> (-81.0306, 25.5)
  line L562 (-80.7461, 26.6191) -> (-81.573, 27.4251)
  line L563 (-81.0306, 25.5) -> (-80.7461, 26.6191)
  line L564 (-79.7956, 25.667) -> (-80.907, 25.3539)
  line L565 (-80.907, 25.3539) -> (-81.1916, 24.2348)
  line L566 (-81.1916, 24.2348) -> (-80.3647, 23.4288)
  line L567 (-80.3647, 23.4288) -> (-79.2532, 23.7419)
  line L568 (-78.9687, 24.861) -> (-79.7956, 25.667)
  line L569 (-79.2532, 23.7419) -> (-78.9687, 24.861)
  line L570 (-78.0182, 23.9089) -> (-79.1296, 23.5958)
  line L571 (-79.1296, 23.5958) -> (-79.4142, 22.4767)
  line L572 (-79.4142, 22.4767) -> (-78.5873, 21.6707)
  line L573 (-78.5873, 21.6707) -> (-77.4758, 21.9838)
  line L574 (-77.1913, 23.1029) -> (-78.0182, 23.9089)
  line L575 (-77.4758, 21.9838) -> (-77.1913, 23.1029)
  line L576 (-76.2408, 22.1508) -> (-77.3522, 21.8377)
  line L577 (-77.3522, 21.8377) -> (-77.6368, 20.7186)
  line L578 (-77.6368, 20.7186) -> (-76.8099, 19.9126)
  line L579 (-76.8099, 19.9126) -> (-75.6984, 20.2257)
  line L580 (-75.4139, 21.3448) -> (-76.2408, 22.1508)
  line L581 (-75.6984, 20.2257) -> (-75.4139, 21.3448)
  line L582 (-74.4634, 20.3927) -> (-75.5748, 20.0796)
  line L583 (-75.5748, 20.0796) -> (-75.8594, 18.9605)
  line L584 (-75.8594, 18.9605) -> (-75.0325, 18.1545)
  line L585 (-75.0325, 18.1545) -> (-73.9211, 18.4676)
  line L586 (-73.6365, 19.5867) -> (-74.4634, 20.3927)
  line L587 (-73.9211, 18.4676) -> (-73.6365, 19.5867)
  line L588 (-72.686, 18.6346) -> (-73.7974, 18.3215)
  line L589 (-73.7974, 18.3215) -> (-74.082, 17.2024)
  line L590 (-74.082, 17.2024) -> (-73.2551, 16.3964)
  line L591 (-73.2551, 16.3964) -> (-72.1437, 16.7096)
  line L592 (-71.8591, 17.8286) -> (-72.686, 18.6346)
  line L593 (-72.1437, 16.7096) -> (-71.8591, 17.8286)
  line L594 (-70.9086, 16.8765) -> (-72.02, 16.5634)
  line L595 (-72.02, 16.5634) -> (-72.3046, 15.4443)
  line L596 (-72.3046, 15.4443) -> (-71.4777, 14.6383)
  line L597 (-71.4777, 14.6383) -> (-70.3663, 14.9515)
  line L598 (-70.0817, 16.0706) -> (-70.9086, 16.8765)
  line L599 (-70.3663, 14.9515) -> (-70.0817, 16.0706)
  line L600 (-69.1312, 15.1184) -> (-70.2426, 14.8053)
  line L601 (-70.2426, 14.8053) -> (-70.5272, 13.6862)
  line L602 (-70.5272, 13.6862) -> (-69.7003, 12.8803)
  line L603 (-69.7003, 12.8803) -> (-68.5889, 13.1934)
  line L604 (-68.3043, 14.3125) -> (-69.1312, 15.1184)
  line L605 (-68.5889, 13.1934) -> (-68.3043, 14.3125)
  line L606 (-67.3538, 13.3604) -> (-68.4652, 13.0472)
  line L607 (-68.4652, 13.0472) -> (-68.7498, 11.9282)
  line L608 (-68.7498, 11.9282) -> (-67.9229, 11.1222)
  line L609 (-67.9229, 11.1222) -> (-66.8115, 11.4353)
  line L610 (-66.5269, 12.5544) -> (-67.3538, 13.3604)
  line L611 (-66.8115, 11.4353) -> (-66.5269, 12.5544)
  line L612 (-65.5764, 11.6023) -> (-66.6878, 11.2892)
  line L613 (-66.6878, 11.2892) -> (-66.9724, 10.1701)
  line L614 (-66.9724, 10.1701) -> (-66.1455, 9.3641)
  line L615 (-66.1455, 9.3641) -> (-65.0341, 9.6772)
  line L616 (-64.7495, 10.7963) -> (-65.5764, 11.6023)
  line L617 (-65.0341, 9.6772) -> (-64.7495, 10.7963)
  line L618 (-81.5923, 30.9605) -> (-82.7037, 30.6474)
  line L619 (-82.7037, 30.6474) -> (-82.9882, 29.5283)
  line L620 (-82.9882, 29.5283) -> (-82.1614, 28.7224)
  line L621 (-82.1614, 28.7224) -> (-81.0499, 29.0355)
  line L622 (-80.7654, 30.1546) -> (-81.5923, 30.9605)
  line L623 (-81.0499, 29.0355) -> (-80.7654, 30.1546)
  line L624 (-79.8149, 29.2024) -> (-80.9263, 28.8893)
  line L625 (-80.9263, 28.8893) -> (-81.2109, 27.7702)
  line L626 (-81.2109, 27.7702) -> (-80.384, 26.9643)
  line L627 (-80.384, 26.9643) -> (-79.2725, 27.2774)
  line L628 (-78.988, 28.3965) -> (-79.8149, 29.2024)
  line L629 (-79.2725, 27.2774) -> (-78.988, 28.3965)
  line L630 (-78.0375, 27.4444) -> (-79.1489, 27.1312)
  line L631 (-79.1489, 27.1312) -> (-79.4335, 26.0122)
  line L632 (-79.4335, 26.0122) -> (-78.6066, 25.2062)
  line L633 (-78.6066, 25.2062) -> (-77.4951, 25.5193)
  line L634 (-77.2106, 26.6384) -> (-78.0375, 27.4444)
  line L635 (-77.4951, 25.5193) -> (-77.2106, 26.6384)
  line L636 (-76.2601, 25.6863) -> (-77.3715, 25.3732)
  line L637 (-77.3715, 25.3732) -> (-77.6561, 24.2541)
  line L638 (-77.6561, 24.2541) -> (-76.8292, 23.4481)
  line L639 (-76.8292, 23.4481) -> (-75.7177, 23.7612)
  line L640 (-75.4332, 24.8803) -> (-76.2601, 25.6863)
  line L641 (-75.7177, 23.7612) -> (-75.4332, 24.8803)
  line L642 (-74.4827, 23.9282) -> (-75.5941, 23.6151)
  line L643 (-75.5941, 23.6151) -> (-75.8787, 22.496)
  line L644 (-75.8787, 22.496) -> (-75.0518, 21.69)
  line L645 (-75.0518, 21.69) -> (-73.9404, 22.0031)
  line L646 (-73.6558, 23.1222) -> (-74.4827, 23.9282)
  line L647 (-73.9404, 22.0031) -> (-73.6558, 23.1222)
  line L648 (-72.7053, 22.1701) -> (-73.8167, 21.857)
  line L649 (-73.8167, 21.857) -> (-74.1013, 20.7379)
  line L650 (-74.1013, 20.7379) -> (-73.2744, 19.9319)
  line L651 (-73.2744, 19.9319) -> (-72.163, 20.245)
  line L652 (-71.8784, 21.3641) -> (-72.7053, 22.1701)
  line L653 (-72.163, 20.245) -> (-71.8784, 21.3641)
  line L654 (-70.9279, 20.412) -> (-72.0393, 20.0989)
  line L655 (-72.0393, 20.0989) -> (-72.3239, 18.9798)
  line L656 (-72.3239, 18.9798) -> (-71.497, 18.1738)
  line L657 (-71.497, 18.1738) -> (-70.3856, 18.4869)
  line L658 (-70.101, 19.606) -> (-70.9279, 20.412)
  line L659 (-70.3856, 18.4869) -> (-70.101, 19.606)
  line L660 (-69.1505, 18.6539) -> (-70.2619, 18.3408)
  line L661 (-70.2619, 18.3408) -> (-70.5465, 17.2217)
  line L662 (-70.5465, 17.2217) -> (-69.7196, 16.4157)
  line L663 (-69.7196, 16.4157) -> (-68.6082, 16.7289)
  line L664 (-68.3236, 17.8479) -> (-69.1505, 18.6539)
  line L665 (-68.6082, 16.7289) -> (-68.3236, 17.8479)
  line L666 (-67.3731, 16.8958) -> (-68.4845, 16.5827)
  line L667 (-68.4845, 16.5827) -> (-68.7691, 15.4636)
  line L668 (-68.7691, 15.4636) -> (-67.9422, 14.6577)
  line L669 (-67.9422, 14.6577) -> (-66.8308, 14.9708)
  line L670 (-66.5462, 16.0899) -> (-67.3731, 16.8958)
  line L671 (-66.8308, 14.9708) -> (-66.5462, 16.0899)
  line L672 (-65.5957, 15.1377) -> (-66.7072, 14.8246)
  line L673 (-66.7072, 14.8246) -> (-66.9917, 13.7055)
  line L674 (-66.9917, 13.7055) -> (-66.1648, 12.8996)
  line L675 (-66.1648, 12.8996) -> (-65.0534, 13.2127)
  line L676 (-64.7688, 14.3318) -> (-65.5957, 15.1377)
  line L677 (-65.0534, 13.2127) -> (-64.7688, 14.3318)
  line L678 (-63.8183, 13.3797) -> (-64.9298, 13.0665)
  line L679 (-64.9298, 13.0665) -> (-65.2143, 11.9475)
  line L680 (-65.2143, 11.9475) -> (-64.3874, 11.1415)
  line L681 (-64.3874, 11.1415) -> (-63.276, 11.4546)
  line L682 (-62.9914, 12.5737) -> (-63.8183, 13.3797)
  line L683 (-63.276, 11.4546) -> (-62.9914, 12.5737)
  line L684 (-79.8342, 32.7379) -> (-80.9456, 32.4248)
  line L685 (-80.9456, 32.4248) -> (-81.2302, 31.3057)
  line L686 (-81.2302, 31.3057) -> (-80.4033, 30.4998)
  line L687 (-80.4033, 30.4998) -> (-79.2918, 30.8129)
  line L688 (-79.0073, 31.932) -> (-79.8342, 32.7379)
  line L689 (-79.2918, 30.8129) -> (-79.0073, 31.932)
  line L690 (-78.0568, 30.9798) -> (-79.1682, 30.6667)
  line L691 (-79.1682, 30.6667) -> (-79.4528, 29.5476)
  line L692 (-79.4528, 29.5476) -> (-78.6259, 28.7417)
  line L693 (-78.6259, 28.7417) -> (-77.5144, 29.0548)
  line L694 (-77.2299, 30.1739) -> (-78.0568, 30.9798)
  line L695 (-77.5144, 29.0548) -> (-77.2299, 30.1739)
  line L696 (-76.2794, 29.2218) -> (-77.3908, 28.9086)
  line L697 (-77.3908, 28.9086) -> (-77.6754, 27.7896)
  line L698 (-77.6754, 27.7896) -> (-76.8485, 26.9836)
  line L699 (-76.8485, 26.9836) -> (-75.7371, 27.2967)
  line L700 (-75.4525, 28.4158) -> (-76.2794, 29.2218)
  line L701 (-75.7371, 27.2967) -> (-75.4525, 28.4158)
  line L702 (-74.502, 27.4637) -> (-75.6134, 27.1506)
  line L703 (-75.6134, 27.1506) -> (-75.898, 26.0315)
  line L704 (-75.898, 26.0315) -> (-75.0711, 25.2255)
  line L705 (-75.0711, 25.2255) -> (-73.9597, 25.5386)
  line L706 (-73.6751, 26.6577) -> (-74.502, 27.4637)
  line L707 (-73.9597, 25.5386) -> (-73.6751, 26.6577)
  line L708 (-72.7246, 25.7056) -> (-73.836, 25.3925)
  line L709 (-73.836, 25.3925) -> (-74.1206, 24.2734)
  line L710 (-74.1206, 24.2734) -> (-73.2937, 23.4674)
  line L711 (-73.2937, 23.4674) -> (-72.1823, 23.7805)
  line L712 (-71.8977, 24.8996) -> (-72.7246, 25.7056)
  line L713 (-72.1823, 23.7805) -> (-71.8977, 24.8996)
  line L714 (-70.9472, 23.9475) -> (-72.0586, 23.6344)
  line L715 (-72.0586, 23.6344) -> (-72.3432, 22.5153)
  line L716 (-72.3432, 22.5153) -> (-71.5163, 21.7093)
  line L717 (-71.5163, 21.7093) -> (-70.4049, 22.0224)
  line L718 (-70.1203, 23.1415) -> (-70.9472, 23.9475)
  line L719 (-70.4049, 22.0224) -> (-70.1203, 23.1415)
  line L720 (-69.1698, 22.1894) -> (-70.2812, 21.8763)
  line L721 (-70.2812, 21.8763) -> (-70.5658, 20.7572)
  line L722 (-70.5658, 20.7572) -> (-69.7389, 19.9512)
  line L723 (-69.7389, 19.9512) -> (-68.6275, 20.2643)
  line L724 (-68.3429, 21.3834) -> (-69.1698, 22.1894)
  line L725 (-68.6275, 20.2643) -> (-68.3429, 21.3834)
  line L726 (-67.3924, 20.4313) -> (-68.5039, 20.1182)
  line L727 (-68.5039, 20.1182) -> (-68.7884, 18.9991)
  line L728 (-68.7884, 18.9991) -> (-67.9615, 18.1931)
  line L729 (-67.9615, 18.1931) -> (-66.8501, 18.5062)
  line L730 (-66.5655, 19.6253) -> (-67.3924, 20.4313)
  line L731 (-66.8501, 18.5062) -> (-66.5655, 19.6253)
  line L732 (-65.615, 18.6732) -> (-66.7265, 18.3601)
  line L733 (-66.7265, 18.3601) -> (-67.011, 17.241)
  line L734 (-67.011, 17.241) -> (-66.1841, 16.435)
  line L735 (-66.1841, 16.435) -> (-65.0727, 16.7482)
  line L736 (-64.7881, 17.8673) -> (-65.615, 18.6732)
  line L737 (-65.0727, 16.7482) -> (-64.7881, 17.8673)
  line L738 (-63.8376, 16.9151) -> (-64.9491, 16.602)
  line L739 (-64.9491, 16.602) -> (-65.2336, 15.4829)
  line L740 (-65.2336, 15.4829) -> (-64.4067, 14.677)
  line L741 (-64.4067, 14.677) -> (-63.2953, 14.9901)
  line L742 (-63.0107, 16.1092) -> (-63.8376, 16.9151)
  line L743 (-63.2953, 14.9901) -> (-63.0107, 16.1092)
  line L744 (-62.0602, 15.1571) -> (-63.1717, 14.8439)
  line L745 (-63.1717, 14.8439) -> (-63.4562, 13.7248)
  line L746 (-63.4562, 13.7248) -> (-62.6293, 12.9189)
  line L747 (-62.6293, 12.9189) -> (-61.5179, 13.232)
  line L748 (-61.2334, 14.3511) -> (-62.0602, 15.1571)
  line L749 (-61.5179, 13.232) -> (-61.2334, 14.3511)
  point P0 (-87, 22)
  point P1 (-80.0222, 13.9414)
  dimension "d99" = 1
  dimension "d102" = 2.5
  dimension "d103" = 2.5
  constraint coincident L4.end L5.start
  constraint coincident L2 L7.end
  constraint perpendicular L2 L7
  constraint coincident L1.end L2.start
  constraint coincident L0.end L1.start
  constraint coincident L0.start L6.end
  constraint coincident L5.end L6.start
  constraint parallel L12 L13
  constraint parallel L7 L14
  constraint parallel L8 L15
  constraint parallel L15 L17
  constraint perpendicular L17 L18
  constraint parallel L10 L16
  constraint parallel L11 L19
  constraint perpendicular L17 L21
  constraint parallel L9 L20
  constraint coincident L5 L23.start
  constraint coincident L4 L22.start
  measures "d99" distance of P1 L29